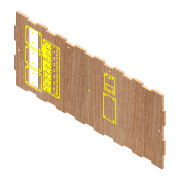
# Autodesk Inventor part: onderplaat elektrobix v2
Saved by Autodesk Inventor 2020.3 (Build 243373000, 373)
## iProperties
Created: 2020-11-25
Part Number: onderplaat elektrobix v2
Material: Wood (Birch)
Document SubType Name: Sheet Metal
Designer: Svend
Density: 0.55 g/cm^3
Sheet Metal Rule: Default_mm
Appearance: Birch - Natural Polished
Author: Svend
Autodesk Inventor part; units mm, degrees
(part 1 of 2)
ref_plane "YZ Plane" through (0, 0, 0) normal (1, 0, 0) x (0, 1, 0)
ref_plane "XZ Plane" through (0, 0, 0) normal (0, 1, 0) x (-1, 0, 0)
ref_plane "XY Plane" through (0, 0, 0) normal (0, 0, 1) x (1, 0, 0)
sketch "Sketch1" plane through (0, 0, 0) normal (0, 0, 1) x (1, 0, 0)
  line L0 (-235, 100) -> (235, 100)
  line L1 (235, 100) -> (235, -100)
  line L2 (235, -100) -> (-235, -100)
  line L3 (-235, -100) -> (-235, 100)
  line L4 (-235, 100) -> (235, -100) construction
  line L5 (235, 100) -> (-235, -100) construction
  line L6 (-15, 94) -> (15, 94)
  line L7 (15, 94) -> (15, 100)
  line L8 (15, 100) -> (-15, 100)
  line L9 (-15, 100) -> (-15, 94)
  line L10 (-15, 94) -> (15, 100) construction
  line L11 (15, 94) -> (-15, 100) construction
  line L12 (45, 94) -> (75, 94)
  line L13 (75, 94) -> (75, 100)
  line L14 (75, 100) -> (45, 100)
  line L15 (45, 100) -> (45, 94)
  line L16 (45, 94) -> (75, 100) construction
  line L17 (75, 94) -> (45, 100) construction
  line L18 (105, 94) -> (135, 94)
  line L19 (135, 94) -> (135, 100)
  line L20 (135, 100) -> (105, 100)
  line L21 (105, 100) -> (105, 94)
  line L22 (105, 94) -> (135, 100) construction
  line L23 (135, 94) -> (105, 100) construction
  line L24 (165, 94) -> (195, 94)
  line L25 (195, 94) -> (195, 100)
  line L26 (195, 100) -> (165, 100)
  line L27 (165, 100) -> (165, 94)
  line L28 (165, 94) -> (195, 100) construction
  line L29 (195, 94) -> (165, 100) construction
  line L30 (-75, 94) -> (-45, 94)
  line L31 (-45, 94) -> (-45, 100)
  line L32 (-45, 100) -> (-75, 100)
  line L33 (-75, 100) -> (-75, 94)
  line L34 (-75, 94) -> (-45, 100) construction
  line L35 (-45, 94) -> (-75, 100) construction
  line L36 (-15, 94) -> (15, 94)
  line L37 (15, 94) -> (15, 100)
  line L38 (15, 100) -> (-15, 100)
  line L39 (-15, 100) -> (-15, 94)
  line L40 (-15, 94) -> (15, 100) construction
  line L41 (15, 94) -> (-15, 100) construction
  line L42 (45, 94) -> (75, 94)
  line L43 (75, 94) -> (75, 100)
  line L44 (75, 100) -> (45, 100)
  line L45 (45, 100) -> (45, 94)
  line L46 (45, 94) -> (75, 100) construction
  line L47 (75, 94) -> (45, 100) construction
  line L48 (105, 94) -> (135, 94)
  line L49 (135, 94) -> (135, 100)
  line L50 (135, 100) -> (105, 100)
  line L51 (105, 100) -> (105, 94)
  line L52 (105, 94) -> (135, 100) construction
  line L53 (135, 94) -> (105, 100) construction
  line L54 (-135, 94) -> (-105, 94)
  line L55 (-105, 94) -> (-105, 100)
  line L56 (-105, 100) -> (-135, 100)
  line L57 (-135, 100) -> (-135, 94)
  line L58 (-135, 94) -> (-105, 100) construction
  line L59 (-105, 94) -> (-135, 100) construction
  line L60 (-75, 94) -> (-45, 94)
  line L61 (-45, 94) -> (-45, 100)
  line L62 (-45, 100) -> (-75, 100)
  line L63 (-75, 100) -> (-75, 94)
  line L64 (-75, 94) -> (-45, 100) construction
  line L65 (-45, 94) -> (-75, 100) construction
  line L66 (-15, 94) -> (15, 94)
  line L67 (15, 94) -> (15, 100)
  line L68 (15, 100) -> (-15, 100)
  line L69 (-15, 100) -> (-15, 94)
  line L70 (-15, 94) -> (15, 100) construction
  line L71 (15, 94) -> (-15, 100) construction
  line L72 (45, 94) -> (75, 94)
  line L73 (75, 94) -> (75, 100)
  line L74 (75, 100) -> (45, 100)
  line L75 (45, 100) -> (45, 94)
  line L76 (45, 94) -> (75, 100) construction
  line L77 (75, 94) -> (45, 100) construction
  line L78 (-195, 94) -> (-165, 94)
  line L79 (-165, 94) -> (-165, 100)
  line L80 (-165, 100) -> (-195, 100)
  line L81 (-195, 100) -> (-195, 94)
  line L82 (-195, 94) -> (-165, 100) construction
  line L83 (-165, 94) -> (-195, 100) construction
  line L84 (-135, 94) -> (-105, 94)
  line L85 (-105, 94) -> (-105, 100)
  line L86 (-105, 100) -> (-135, 100)
  line L87 (-135, 100) -> (-135, 94)
  line L88 (-135, 94) -> (-105, 100) construction
  line L89 (-105, 94) -> (-135, 100) construction
  line L90 (-75, 94) -> (-45, 94)
  line L91 (-45, 94) -> (-45, 100)
  line L92 (-45, 100) -> (-75, 100)
  line L93 (-75, 100) -> (-75, 94)
  line L94 (-75, 94) -> (-45, 100) construction
  line L95 (-45, 94) -> (-75, 100) construction
  line L96 (-15, 94) -> (15, 94)
  line L97 (15, 94) -> (15, 100)
  line L98 (15, 100) -> (-15, 100)
  line L99 (-15, 100) -> (-15, 94)
  line L100 (-15, 94) -> (15, 100) construction
  line L101 (15, 94) -> (-15, 100) construction
  line L102 (229, -20) -> (235, -20)
  line L103 (235, -20) -> (235, 20)
  line L104 (235, 20) -> (229, 20)
  line L105 (229, 20) -> (229, -20)
  line L106 (229, -20) -> (235, 20) construction
  line L107 (235, -20) -> (229, 20) construction
  line L108 (235, 100) -> (229, 100)
  line L109 (229, 100) -> (229, 60)
  line L110 (229, 60) -> (235, 60)
  line L111 (235, 60) -> (235, 100)
  line L112 (235, -100) -> (229, -100)
  line L113 (229, -100) -> (229, -60)
  line L114 (229, -60) -> (235, -60)
  line L115 (235, -60) -> (235, -100)
  line L116 (0, 100) -> (0, -100) construction
  line L117 (235, 0) -> (-235, 0) construction
  line L118 (-229, -20) -> (-235, -20)
  line L119 (-235, -20) -> (-235, 20)
  line L120 (-235, 20) -> (-229, 20)
  line L121 (-229, 20) -> (-229, -20)
  line L122 (-229, -20) -> (-235, 20) construction
  line L123 (-235, -20) -> (-229, 20) construction
  line L124 (-235, 100) -> (-229, 100)
  line L125 (-229, 100) -> (-229, 60)
  line L126 (-229, 60) -> (-235, 60)
  line L127 (-235, 60) -> (-235, 100)
  line L128 (-235, -100) -> (-229, -100)
  line L129 (-229, -100) -> (-229, -60)
  line L130 (-229, -60) -> (-235, -60)
  line L131 (-235, -60) -> (-235, -100)
  line L132 (-15, -94) -> (15, -94)
  line L133 (15, -94) -> (15, -100)
  line L134 (15, -100) -> (-15, -100)
  line L135 (-15, -100) -> (-15, -94)
  line L136 (-15, -94) -> (15, -100) construction
  line L137 (15, -94) -> (-15, -100) construction
  line L138 (45, -100) -> (45, -94)
  line L139 (45, -94) -> (75, -94)
  line L140 (75, -100) -> (45, -100)
  line L141 (45, -94) -> (75, -100) construction
  line L142 (75, -94) -> (45, -100) construction
  line L143 (75, -94) -> (75, -100)
  line L144 (105, -100) -> (105, -94)
  line L145 (105, -94) -> (135, -94)
  line L146 (135, -100) -> (105, -100)
  line L147 (105, -94) -> (135, -100) construction
  line L148 (135, -94) -> (105, -100) construction
  line L149 (135, -94) -> (135, -100)
  line L150 (165, -100) -> (165, -94)
  line L151 (165, -94) -> (195, -94)
  line L152 (195, -100) -> (165, -100)
  line L153 (165, -94) -> (195, -100) construction
  line L154 (195, -94) -> (165, -100) construction
  line L155 (195, -94) -> (195, -100)
  line L156 (-75, -100) -> (-75, -94)
  line L157 (-75, -94) -> (-45, -94)
  line L158 (-45, -100) -> (-75, -100)
  line L159 (-75, -94) -> (-45, -100) construction
  line L160 (-45, -94) -> (-75, -100) construction
  line L161 (-45, -94) -> (-45, -100)
  line L162 (-15, -100) -> (-15, -94)
  line L163 (-15, -94) -> (15, -94)
  line L164 (15, -100) -> (-15, -100)
  line L165 (-15, -94) -> (15, -100) construction
  line L166 (15, -94) -> (-15, -100) construction
  line L167 (15, -94) -> (15, -100)
  line L168 (45, -100) -> (45, -94)
  line L169 (45, -94) -> (75, -94)
  line L170 (75, -100) -> (45, -100)
  line L171 (45, -94) -> (75, -100) construction
  line L172 (75, -94) -> (45, -100) construction
  line L173 (75, -94) -> (75, -100)
  line L174 (105, -100) -> (105, -94)
  line L175 (105, -94) -> (135, -94)
  line L176 (135, -100) -> (105, -100)
  line L177 (105, -94) -> (135, -100) construction
  line L178 (135, -94) -> (105, -100) construction
  line L179 (135, -94) -> (135, -100)
  line L180 (-135, -100) -> (-135, -94)
  line L181 (-135, -94) -> (-105, -94)
  line L182 (-105, -100) -> (-135, -100)
  line L183 (-135, -94) -> (-105, -100) construction
  line L184 (-105, -94) -> (-135, -100) construction
  line L185 (-105, -94) -> (-105, -100)
  line L186 (-75, -100) -> (-75, -94)
  line L187 (-75, -94) -> (-45, -94)
  line L188 (-45, -100) -> (-75, -100)
  line L189 (-75, -94) -> (-45, -100) construction
  line L190 (-45, -94) -> (-75, -100) construction
  line L191 (-45, -94) -> (-45, -100)
  line L192 (-15, -100) -> (-15, -94)
  line L193 (-15, -94) -> (15, -94)
  line L194 (15, -100) -> (-15, -100)
  line L195 (-15, -94) -> (15, -100) construction
  line L196 (15, -94) -> (-15, -100) construction
  line L197 (15, -94) -> (15, -100)
  line L198 (45, -100) -> (45, -94)
  line L199 (45, -94) -> (75, -94)
  line L200 (75, -100) -> (45, -100)
  line L201 (45, -94) -> (75, -100) construction
  line L202 (75, -94) -> (45, -100) construction
  line L203 (75, -94) -> (75, -100)
  line L204 (-195, -100) -> (-195, -94)
  line L205 (-195, -94) -> (-165, -94)
  line L206 (-165, -100) -> (-195, -100)
  line L207 (-195, -94) -> (-165, -100) construction
  line L208 (-165, -94) -> (-195, -100) construction
  line L209 (-165, -94) -> (-165, -100)
  line L210 (-135, -100) -> (-135, -94)
  line L211 (-135, -94) -> (-105, -94)
  line L212 (-105, -100) -> (-135, -100)
  line L213 (-135, -94) -> (-105, -100) construction
  line L214 (-105, -94) -> (-135, -100) construction
  line L215 (-105, -94) -> (-105, -100)
  line L216 (-75, -100) -> (-75, -94)
  line L217 (-75, -94) -> (-45, -94)
  line L218 (-45, -100) -> (-75, -100)
  line L219 (-75, -94) -> (-45, -100) construction
  line L220 (-45, -94) -> (-75, -100) construction
  line L221 (-45, -94) -> (-45, -100)
  line L222 (-15, -100) -> (-15, -94)
  line L223 (-15, -94) -> (15, -94)
  line L224 (15, -100) -> (-15, -100)
  line L225 (-15, -94) -> (15, -100) construction
  line L226 (15, -94) -> (-15, -100) construction
  line L227 (15, -94) -> (15, -100)
  circle A0 centre (-65, 85) radius 3
  circle A1 centre (65, 85) radius 3
  line L228 (65, 85) -> (-65, 85) construction
  circle A2 centre (-220, 0) radius 3
  circle A3 centre (220, 0) radius 3
  point P0 (0, 0)
  point P1 (0, 97)
  point P2 (0, 97)
  point P3 (0, 0)
  point P4 (60, 97)
  point P5 (60, 97)
  point P6 (120, 97)
  point P7 (120, 97)
  point P8 (180, 97)
  point P9 (180, 97)
  point P10 (-60, 97)
  point P11 (-60, 97)
  point P12 (0, 97)
  point P13 (0, 97)
  point P14 (60, 97)
  point P15 (60, 97)
  point P16 (120, 97)
  point P17 (120, 97)
  point P18 (-120, 97)
  point P19 (-120, 97)
  point P20 (-60, 97)
  point P21 (-60, 97)
  point P22 (0, 97)
  point P23 (0, 97)
  point P24 (60, 97)
  point P25 (60, 97)
  point P26 (-180, 97)
  point P27 (-180, 97)
  point P28 (-120, 97)
  point P29 (-120, 97)
  point P30 (-60, 97)
  point P31 (-60, 97)
  point P32 (0, 97)
  point P33 (0, 97)
  point P34 (232, 0)
  point P35 (232, 0)
  point P36 (0, 0)
  point P37 (-232, 0)
  point P38 (-232, 0)
  point P39 (0, -97)
  point P40 (60, -100)
  point P41 (60, -97)
  point P42 (120, -100)
  point P43 (120, -97)
  point P44 (180, -100)
  point P45 (180, -97)
  point P46 (-60, -100)
  point P47 (-60, -97)
  point P48 (0, -97)
  point P49 (60, -100)
  point P50 (60, -97)
  point P51 (120, -100)
  point P52 (120, -97)
  point P53 (-120, -100)
  point P54 (-120, -97)
  point P55 (-60, -100)
  point P56 (-60, -97)
  point P57 (0, -97)
  point P58 (60, -100)
  point P59 (60, -97)
  point P60 (-180, -100)
  point P61 (-180, -97)
  point P62 (-120, -100)
  point P63 (-120, -97)
  point P64 (-60, -100)
  point P65 (-60, -97)
  point P66 (0, -97)
  point P67 (0, 85)
  point P68 (0, 100)
  dimension "d0" = 470
  dimension "d1" = 200
  dimension "d2" = 6
  dimension "d3" = 30
  dimension "d6" = 60
  dimension "d9" = 60
  dimension "d12" = 6
  dimension "d13" = 40
  dimension "d14" = 6
  dimension "d15" = 40
  dimension "d16" = 6
  dimension "d17" = 40
  dimension "d20" = 60
  dimension "d23" = 60
  dimension "d26" = 6
  dimension "d27" = 15
  dimension "d28" = 130
  dimension "d29" = 6
  dimension "d30" = 6
  dimension "d31" = 15
  dimension "d32" = 15
  measures "d0" distance of L1.end L2.end
  measures "d1" distance of L0.end L1.end
  measures "d2" distance of L6.end L7.end
  measures "d3" distance of L6.start L6.end
  measures "d6" distance of L6.start L12.start
  measures "d9" distance of L6.start L30.start
  measures "d12" distance of L103.end L104.end
  measures "d13" distance of L104.end L102.start
  measures "d14" distance of L110.end L109.end
  measures "d15" distance of L109.end L108.end
  measures "d16" distance of L113.end L114.end
  measures "d17" distance of L112.end L113.end
  measures "d20" distance of L116.end point (60, -100)
  measures "d23" distance of L116.end point (-60, -100)
  measures "d26" diameter of A1
  measures "d27" distance between parallel lines of L0 L228
  measures "d28" distance of L228.start L228.end
  measures "d29" diameter of A2
  measures "d30" diameter of A3
  measures "d31" distance from line of L3 A2.centre
  measures "d32" distance from line of L103 A3.centre
extrude "Plate1" add sketch "Sketch1" along normal blind 6 contours L0 L81 L78 L79 L57 L54 L55 L33 L30 L31 L9 L6 L7 L15 L12 L13 L21 L18 L19 L27 L24 L25 L109 L110 L1 L104 L105 L102 L114 L113 L2 L155 L151 L150 L149 L145 L144 L143 L139 L138 L133 L132 L135 L161 L157 L156 L185 L181 L180 L209 L205 L204 L129 L130 L3 L118 L121 L120 L126 L125
sketch "Sketch2" plane through (0, 0, 0) normal (0, 0, -1) x (-1, 0, 0)
  line L0 (160, -80) -> (193, -80)
  line L1 (193, -80) -> (193, 80)
  line L2 (193, 80) -> (160, 80)
  line L3 (160, 80) -> (160, -80)
  circle A0 centre (65, 85) radius 3 projected
  circle A1 centre (-65, 85) radius 3 projected
  circle A2 centre (220, 0) radius 3 projected
  circle A3 centre (-220, 0) radius 3 projected
  line L4 (235, -20) -> (229, -20) projected
  line L5 (229, -20) -> (229, 20) projected
  line L6 (229, 20) -> (235, 20) projected
  line L7 (235, 60) -> (235, 20) projected
  line L8 (235, 60) -> (229, 60) projected
  line L9 (229, 60) -> (229, 100) projected
  line L10 (195, 100) -> (229, 100) projected
  line L11 (195, 100) -> (195, 94) projected
  line L12 (195, 94) -> (165, 94) projected
  line L13 (165, 94) -> (165, 100) projected
  line L14 (135, 100) -> (165, 100) projected
  line L15 (135, 100) -> (135, 94) projected
  line L16 (135, 94) -> (105, 94) projected
  line L17 (105, 94) -> (105, 100) projected
  line L18 (75, 100) -> (105, 100) projected
  line L19 (75, 100) -> (75, 94) projected
  line L20 (75, 94) -> (45, 94) projected
  line L21 (45, 94) -> (45, 100) projected
  line L22 (15, 100) -> (45, 100) projected
  line L23 (15, 100) -> (15, 94) projected
  line L24 (15, 94) -> (-15, 94) projected
  line L25 (-15, 94) -> (-15, 100) projected
  line L26 (-45, 100) -> (-15, 100) projected
  line L27 (-45, 100) -> (-45, 94) projected
  line L28 (-45, 94) -> (-75, 94) projected
  line L29 (-75, 94) -> (-75, 100) projected
  line L30 (-105, 100) -> (-75, 100) projected
  line L31 (-105, 100) -> (-105, 94) projected
  line L32 (-105, 94) -> (-135, 94) projected
  line L33 (-135, 94) -> (-135, 100) projected
  line L34 (-165, 100) -> (-135, 100) projected
  line L35 (-165, 100) -> (-165, 94) projected
  line L36 (-165, 94) -> (-195, 94) projected
  line L37 (-195, 94) -> (-195, 100) projected
  line L38 (-229, 100) -> (-195, 100) projected
  line L39 (-229, 100) -> (-229, 60) projected
  line L40 (-229, 60) -> (-235, 60) projected
  line L41 (-235, 20) -> (-235, 60) projected
  line L42 (-235, 20) -> (-229, 20) projected
  line L43 (-229, 20) -> (-229, -20) projected
  line L44 (-229, -20) -> (-235, -20) projected
  line L45 (-235, -60) -> (-235, -20) projected
  line L46 (-235, -60) -> (-229, -60) projected
  line L47 (-229, -60) -> (-229, -100) projected
  line L48 (-195, -100) -> (-229, -100) projected
  line L49 (-195, -100) -> (-195, -94) projected
  line L50 (-195, -94) -> (-165, -94) projected
  line L51 (-165, -94) -> (-165, -100) projected
  line L52 (-135, -100) -> (-165, -100) projected
  line L53 (-135, -100) -> (-135, -94) projected
  line L54 (-135, -94) -> (-105, -94) projected
  line L55 (-105, -94) -> (-105, -100) projected
  line L56 (-75, -100) -> (-105, -100) projected
  line L57 (-75, -100) -> (-75, -94) projected
  line L58 (-75, -94) -> (-45, -94) projected
  line L59 (-45, -94) -> (-45, -100) projected
  line L60 (-15, -100) -> (-45, -100) projected
  line L61 (-15, -100) -> (-15, -94) projected
  line L62 (-15, -94) -> (15, -94) projected
  line L63 (15, -94) -> (15, -100) projected
  line L64 (45, -100) -> (15, -100) projected
  line L65 (45, -100) -> (45, -94) projected
  line L66 (45, -94) -> (75, -94) projected
  line L67 (75, -94) -> (75, -100) projected
  line L68 (105, -100) -> (75, -100) projected
  line L69 (105, -100) -> (105, -94) projected
  line L70 (105, -94) -> (135, -94) projected
  line L71 (135, -94) -> (135, -100) projected
  line L72 (165, -100) -> (135, -100) projected
  line L73 (165, -100) -> (165, -94) projected
  line L74 (165, -94) -> (195, -94) projected
  line L75 (195, -94) -> (195, -100) projected
  line L76 (229, -100) -> (195, -100) projected
  line L77 (229, -100) -> (229, -60) projected
  line L78 (229, -60) -> (235, -60) projected
  line L79 (235, -20) -> (235, -60) projected
  point P0 (0, 0)
  point P1 (193, 0)
  point P2 (229, 0)
  dimension "d34" = 33
  dimension "d35" = 160
  dimension "d36" = 36
  constraints: 8 end point, 2 midpoint, 2 parallel, 1 horizontal, 1 horizontal alignment, 1 perpendicular
  measures "d34" distance of L2.end L1.end
  measures "d35" distance of L1.end L0.end
  measures "d36" distance between parallel lines of L5 L1
extrude "Cut1" cut sketch "Sketch2" against normal blind 6 contours L3 L2 L1 L0
sketch "Sketch3" plane through (0, 0, 6) normal (0, 0, 1) x (1, 0, 0)
  line L0 (-153.2, -29.5) -> (-195, -29.5)
  line L1 (-195, -29.5) -> (-199, -33.5)
  line L2 (-199, -33.5) -> (-199, -75)
  line L3 (-199, -75) -> (-195, -79)
  line L4 (-195, -79) -> (-153.2, -79)
  line L5 (-153.2, -79) -> (-149.2, -75)
  line L6 (-149.2, -75) -> (-149.2, -33.5)
  line L7 (-149.2, -33.5) -> (-153.2, -29.5)
  circle A0 centre (-176.5, -40.75) radius 1.6
  circle A1 centre (-176.5, -67.75) radius 1.6
  circle A2 centre (-195.4, -34.25) radius 1.6
  circle A3 centre (-195.4, -74.25) radius 1.6
  circle A4 centre (-155.4, -74.25) radius 1.6
  circle A5 centre (-155.4, -34.25) radius 1.6
  line L8 (-153.2, 25) -> (-195, 25)
  line L9 (-195, 25) -> (-199, 21)
  line L10 (-199, 21) -> (-199, -20.5)
  line L11 (-199, -20.5) -> (-195, -24.5)
  line L12 (-195, -24.5) -> (-153.2, -24.5)
  line L13 (-153.2, -24.5) -> (-149.2, -20.5)
  line L14 (-149.2, -20.5) -> (-149.2, 21)
  line L15 (-149.2, 21) -> (-153.2, 25)
  circle A6 centre (-176.5, 13.75) radius 1.6
  circle A7 centre (-176.5, -13.25) radius 1.6
  circle A8 centre (-195.4, 20.25) radius 1.6
  circle A9 centre (-195.4, -19.75) radius 1.6
  circle A10 centre (-155.4, -19.75) radius 1.6
  circle A11 centre (-155.4, 20.25) radius 1.6
  line L16 (-153.2, 79.5) -> (-195, 79.5)
  line L17 (-195, 79.5) -> (-199, 75.5)
  line L18 (-199, 75.5) -> (-199, 34)
  line L19 (-199, 34) -> (-195, 30)
  line L20 (-195, 30) -> (-153.2, 30)
  line L21 (-153.2, 30) -> (-149.2, 34)
  line L22 (-149.2, 34) -> (-149.2, 75.5)
  line L23 (-149.2, 75.5) -> (-153.2, 79.5)
  circle A12 centre (-176.5, 68.25) radius 1.6
  circle A13 centre (-176.5, 41.25) radius 1.6
  circle A14 centre (-195.4, 74.75) radius 1.6
  circle A15 centre (-195.4, 34.75) radius 1.6
  circle A16 centre (-155.4, 34.75) radius 1.6
  circle A17 centre (-155.4, 74.75) radius 1.6
  arc A18 (-96.55, -69) -> (-94, -66.45) centre (-96.55, -66.45) ccw
  line L24 (-94, -66.45) -> (-94, 66.45)
  arc A19 (-94, 66.45) -> (-96.55, 69) centre (-96.55, 66.45) ccw
  line L25 (-96.55, 69) -> (-141.45, 69)
  arc A20 (-141.45, 69) -> (-144, 66.45) centre (-141.45, 66.45) ccw
  line L26 (-144, 66.45) -> (-144, -66.45)
  arc A21 (-144, -66.45) -> (-141.45, -69) centre (-141.45, -66.45) ccw
  line L27 (-141.45, -69) -> (-96.55, -69)
  line L28 (-137, -48.3571) -> (-137, -42.7571)
  line L29 (-137, -42.7571) -> (-131, -42.7571)
  line L30 (-131, -42.7571) -> (-131, -48.3571)
  line L31 (-131, -48.3571) -> (-137, -48.3571)
  line L32 (-129.5, -38.6571) -> (-129.5, -38.3571)
  line L33 (-129.5, -38.3571) -> (-127.6, -38.3571)
  line L34 (-127.6, -38.3571) -> (-127.6, -37.6571)
  line L35 (-127.6, -37.6571) -> (-127.3, -37.6571)
  line L36 (-127.3, -37.6571) -> (-127.3, -38.6571)
  line L37 (-127.3, -38.6571) -> (-129.5, -38.6571)
  line L38 (-138.3, 8.9714) -> (-138.3, 14.1714)
  line L39 (-138.3, 14.1714) -> (-135.7, 14.1714)
  line L40 (-135.7, 14.1714) -> (-135.7, 8.9714)
  line L41 (-135.7, 8.9714) -> (-138.3, 8.9714)
  line L42 (-128.7, 7.9714) -> (-126, 7.9714)
  line L43 (-126, 7.9714) -> (-126, 10.3714)
  line L44 (-126, 10.3714) -> (-124.2, 12.1714)
  line L45 (-124.2, 12.1714) -> (-119.5, 12.1714)
  line L46 (-119.5, 12.1714) -> (-119.5, 11.0714)
  line L47 (-119.5, 11.0714) -> (-123.8858, 11.0714)
  line L48 (-123.8858, 11.0714) -> (-124.9, 10.0572)
  line L49 (-124.9, 10.0572) -> (-124.9, 6.2856)
  line L50 (-124.9, 6.2856) -> (-123.8858, 5.2714)
  line L51 (-123.8858, 5.2714) -> (-119.5, 5.2714)
  line L52 (-119.5, 5.2714) -> (-119.5, 4.1714)
  line L53 (-119.5, 4.1714) -> (-124.2, 4.1714)
  line L54 (-124.2, 4.1714) -> (-126, 5.9714)
  line L55 (-126, 5.9714) -> (-126, 1.2714)
  line L56 (-126, 1.2714) -> (-128.7, 1.2714)
  line L57 (-128.7, 1.2714) -> (-128.7, 7.9714)
  line L58 (-138.3, 42.0571) -> (-138.3, 47.2571)
  line L59 (-138.3, 47.2571) -> (-135.7, 47.2571)
  line L60 (-135.7, 47.2571) -> (-135.7, 42.0571)
  line L61 (-135.7, 42.0571) -> (-138.3, 42.0571)
  line L62 (-135.5, 47.2571) -> (-133.2, 47.2571)
  line L63 (-133.2, 47.2571) -> (-133.2, 42.0571)
  line L64 (-133.2, 42.0571) -> (-135.5, 42.0571)
  line L65 (-135.5, 42.0571) -> (-135.5, 47.2571)
  line L66 (-128.7, 41.0571) -> (-126, 41.0571)
  line L67 (-126, 41.0571) -> (-126, 43.4571)
  line L68 (-126, 43.4571) -> (-124.2, 45.2571)
  line L69 (-124.2, 45.2571) -> (-119.5, 45.2571)
  line L70 (-119.5, 45.2571) -> (-119.5, 44.1571)
  line L71 (-119.5, 44.1571) -> (-123.8858, 44.1571)
  line L72 (-123.8858, 44.1571) -> (-124.9, 43.1429)
  line L73 (-124.9, 43.1429) -> (-124.9, 39.3714)
  line L74 (-124.9, 39.3714) -> (-123.8858, 38.3571)
  line L75 (-123.8858, 38.3571) -> (-119.5, 38.3571)
  line L76 (-119.5, 38.3571) -> (-119.5, 37.2571)
  line L77 (-119.5, 37.2571) -> (-124.2, 37.2571)
  line L78 (-124.2, 37.2571) -> (-126, 39.0571)
  line L79 (-126, 39.0571) -> (-126, 34.3571)
  line L80 (-126, 34.3571) -> (-128.7, 34.3571)
  line L81 (-128.7, 34.3571) -> (-128.7, 41.0571)
  line L82 (-128.7, 24.5143) -> (-126, 24.5143)
  line L83 (-126, 24.5143) -> (-126, 26.9143)
  line L84 (-126, 26.9143) -> (-124.2, 28.7143)
  line L85 (-124.2, 28.7143) -> (-119.5, 28.7143)
  line L86 (-119.5, 28.7143) -> (-119.5, 27.6143)
  line L87 (-119.5, 27.6143) -> (-123.8858, 27.6143)
  line L88 (-123.8858, 27.6143) -> (-124.9, 26.6001)
  line L89 (-124.9, 26.6001) -> (-124.9, 22.8285)
  line L90 (-124.9, 22.8285) -> (-123.8858, 21.8143)
  line L91 (-123.8858, 21.8143) -> (-119.5, 21.8143)
  line L92 (-119.5, 21.8143) -> (-119.5, 20.7143)
  line L93 (-119.5, 20.7143) -> (-124.2, 20.7143)
  line L94 (-124.2, 20.7143) -> (-126, 22.5143)
  line L95 (-126, 22.5143) -> (-126, 17.8143)
  line L96 (-126, 17.8143) -> (-128.7, 17.8143)
  line L97 (-128.7, 17.8143) -> (-128.7, 24.5143)
  line L98 (-133, 14.1714) -> (-130.7, 14.1714)
  line L99 (-130.7, 14.1714) -> (-130.7, 8.9714)
  line L100 (-130.7, 8.9714) -> (-133, 8.9714)
  line L101 (-133, 8.9714) -> (-133, 14.1714)
  line L102 (-135.5, -18.9143) -> (-133.2, -18.9143)
  line L103 (-133.2, -18.9143) -> (-133.2, -24.1143)
  line L104 (-133.2, -24.1143) -> (-135.5, -24.1143)
  line L105 (-135.5, -24.1143) -> (-135.5, -18.9143)
  line L106 (-133, -52) -> (-130.7, -52)
  line L107 (-130.7, -52) -> (-130.7, -57.2)
  line L108 (-130.7, -57.2) -> (-133, -57.2)
  line L109 (-133, -57.2) -> (-133, -52)
  line L110 (-138.3, -40.6571) -> (-138.3, -35.4571)
  line L111 (-138.3, -35.4571) -> (-135.7, -35.4571)
  line L112 (-135.7, -35.4571) -> (-135.7, -40.6571)
  line L113 (-135.7, -40.6571) -> (-138.3, -40.6571)
  line L114 (-127.3, -35.4571) -> (-127.3, -36.4571)
  line L115 (-127.3, -36.4571) -> (-127.6, -36.4571)
  line L116 (-127.6, -36.4571) -> (-127.6, -35.7571)
  line L117 (-127.6, -35.7571) -> (-129.5, -35.7571)
  line L118 (-129.5, -35.7571) -> (-129.5, -35.4571)
  line L119 (-129.5, -35.4571) -> (-127.3, -35.4571)
  line L120 (-137, -15.2714) -> (-137, -9.6714)
  line L121 (-137, -9.6714) -> (-131, -9.6714)
  line L122 (-131, -9.6714) -> (-131, -15.2714)
  line L123 (-131, -15.2714) -> (-137, -15.2714)
  line L124 (-135.5, 14.1714) -> (-133.2, 14.1714)
  line L125 (-133.2, 14.1714) -> (-133.2, 8.9714)
  line L126 (-133.2, 8.9714) -> (-135.5, 8.9714)
  line L127 (-135.5, 8.9714) -> (-135.5, 14.1714)
  line L128 (-129.5, 10.9714) -> (-129.5, 11.2714)
  line L129 (-129.5, 11.2714) -> (-127.6, 11.2714)
  line L130 (-127.6, 11.2714) -> (-127.6, 11.9714)
  line L131 (-127.6, 11.9714) -> (-127.3, 11.9714)
  line L132 (-127.3, 11.9714) -> (-127.3, 10.9714)
  line L133 (-127.3, 10.9714) -> (-129.5, 10.9714)
  line L134 (-138.3, 63.8) -> (-135.7, 63.8)
  line L135 (-135.7, 63.8) -> (-135.7, 58.6)
  line L136 (-135.7, 58.6) -> (-138.3, 58.6)
  line L137 (-138.3, 58.6) -> (-138.3, 63.8)
  line L138 (-137, 56.5) -> (-131, 56.5)
  line L139 (-131, 56.5) -> (-131, 50.9)
  line L140 (-131, 50.9) -> (-137, 50.9)
  line L141 (-137, 50.9) -> (-137, 56.5)
  line L142 (-127.3, 63.8) -> (-127.3, 62.8)
  line L143 (-127.3, 62.8) -> (-127.6, 62.8)
  line L144 (-127.6, 62.8) -> (-127.6, 63.5)
  line L145 (-127.6, 63.5) -> (-129.5, 63.5)
  line L146 (-129.5, 63.5) -> (-129.5, 63.8)
  line L147 (-129.5, 63.8) -> (-127.3, 63.8)
  line L148 (-137, 34.3571) -> (-137, 39.9571)
  line L149 (-137, 39.9571) -> (-131, 39.9571)
  line L150 (-131, 39.9571) -> (-131, 34.3571)
  line L151 (-131, 34.3571) -> (-137, 34.3571)
  line L152 (-137, 1.2714) -> (-137, 6.8714)
  line L153 (-137, 6.8714) -> (-131, 6.8714)
  line L154 (-131, 6.8714) -> (-131, 1.2714)
  line L155 (-131, 1.2714) -> (-137, 1.2714)
  line L156 (-138.3, -24.1143) -> (-138.3, -18.9143)
  line L157 (-138.3, -18.9143) -> (-135.7, -18.9143)
  line L158 (-135.7, -18.9143) -> (-135.7, -24.1143)
  line L159 (-135.7, -24.1143) -> (-138.3, -24.1143)
  line L160 (-135.5, -52) -> (-133.2, -52)
  line L161 (-133.2, -52) -> (-133.2, -57.2)
  line L162 (-133.2, -57.2) -> (-135.5, -57.2)
  line L163 (-135.5, -57.2) -> (-135.5, -52)
  circle A22 centre (-137.8, -63.36) radius 0.6
  line L164 (-130.3, -53.4) -> (-130.3, -52.5)
  line L165 (-130.3, -52.5) -> (-129.7, -52.5)
  line L166 (-129.7, -52.5) -> (-129.7, -53.4)
  line L167 (-129.7, -53.4) -> (-130.3, -53.4)
  circle A23 centre (-137.8, -44.2771) radius 0.6
  circle A24 centre (-130.18, -30.2743) radius 0.6
  line L168 (-127.9, -20.9643) -> (-127.9, -20.0643)
  line L169 (-127.9, -20.0643) -> (-127.3, -20.0643)
  line L170 (-127.3, -20.0643) -> (-127.3, -20.9643)
  line L171 (-127.3, -20.9643) -> (-127.9, -20.9643)
  circle A25 centre (-130.18, -11.1914) radius 0.6
  line L172 (-130.3, -5.0714) -> (-130.3, -4.1714)
  line L173 (-130.3, -4.1714) -> (-129.7, -4.1714)
  line L174 (-129.7, -4.1714) -> (-129.7, -5.0714)
  line L175 (-129.7, -5.0714) -> (-130.3, -5.0714)
  circle A26 centre (-137.8, 2.8114) radius 0.6
  line L176 (-130.3, 12.7714) -> (-130.3, 13.6714)
  line L177 (-130.3, 13.6714) -> (-129.7, 13.6714)
  line L178 (-129.7, 13.6714) -> (-129.7, 12.7714)
  line L179 (-129.7, 12.7714) -> (-130.3, 12.7714)
  circle A27 centre (-137.8, 21.8943) radius 0.6
  circle A28 centre (-130.18, 35.8971) radius 0.6
  line L180 (-127.9, 45.2071) -> (-127.9, 46.1071)
  line L181 (-127.9, 46.1071) -> (-127.3, 46.1071)
  line L182 (-127.3, 46.1071) -> (-127.3, 45.2071)
  line L183 (-127.3, 45.2071) -> (-127.9, 45.2071)
  circle A29 centre (-137.8, 52.44) radius 0.6
  circle A30 centre (-130.18, 52.44) radius 0.6
  line L184 (-127.3, 61.75) -> (-127.9, 61.75)
  line L185 (-127.9, 61.75) -> (-127.9, 62.65)
  line L186 (-127.9, 62.65) -> (-127.3, 62.65)
  line L187 (-127.3, 62.65) -> (-127.3, 61.75)
  circle A31 centre (-137.8, 38.4371) radius 0.6
  line L188 (-130.3, 29.3143) -> (-130.3, 30.2143)
  line L189 (-130.3, 30.2143) -> (-129.7, 30.2143)
  line L190 (-129.7, 30.2143) -> (-129.7, 29.3143)
  line L191 (-129.7, 29.3143) -> (-130.3, 29.3143)
  circle A32 centre (-137.8, 19.3543) radius 0.6
  line L192 (-130.3, 11.4714) -> (-130.3, 12.3714)
  line L193 (-130.3, 12.3714) -> (-129.7, 12.3714)
  line L194 (-129.7, 12.3714) -> (-129.7, 11.4714)
  line L195 (-129.7, 11.4714) -> (-130.3, 11.4714)
  circle A33 centre (-130.18, 5.3514) radius 0.6
  line L196 (-127.9, -4.4214) -> (-127.9, -3.5214)
  line L197 (-127.9, -3.5214) -> (-127.3, -3.5214)
  line L198 (-127.3, -3.5214) -> (-127.3, -4.4214)
  line L199 (-127.3, -4.4214) -> (-127.9, -4.4214)
  circle A34 centre (-130.18, -13.7314) radius 0.6
  circle A35 centre (-137.8, -27.7343) radius 0.6
  line L200 (-127.9, -37.5071) -> (-127.9, -36.6071)
  line L201 (-127.9, -36.6071) -> (-127.3, -36.6071)
  line L202 (-127.3, -36.6071) -> (-127.3, -37.5071)
  line L203 (-127.3, -37.5071) -> (-127.9, -37.5071)
  circle A36 centre (-137.8, -46.8171) radius 0.6
  line L204 (-130.3, -54.7) -> (-130.3, -53.8)
  line L205 (-130.3, -53.8) -> (-129.7, -53.8)
  line L206 (-129.7, -53.8) -> (-129.7, -54.7)
  line L207 (-129.7, -54.7) -> (-130.3, -54.7)
  circle A37 centre (-130.18, -60.82) radius 0.6
  circle A38 centre (-137.8, -60.82) radius 0.6
  circle A39 centre (-130.18, -46.8171) radius 0.6
  line L208 (-130.3, -38.1571) -> (-130.3, -37.2571)
  line L209 (-130.3, -37.2571) -> (-129.7, -37.2571)
  line L210 (-129.7, -37.2571) -> (-129.7, -38.1571)
  line L211 (-129.7, -38.1571) -> (-130.3, -38.1571)
  circle A40 centre (-130.18, -27.7343) radius 0.6
  line L212 (-130.3, -21.6143) -> (-130.3, -20.7143)
  line L213 (-130.3, -20.7143) -> (-129.7, -20.7143)
  line L214 (-129.7, -20.7143) -> (-129.7, -21.6143)
  line L215 (-129.7, -21.6143) -> (-130.3, -21.6143)
  circle A41 centre (-137.8, -13.7314) radius 0.6
  line L216 (-130.3, -3.7714) -> (-130.3, -2.8714)
  line L217 (-130.3, -2.8714) -> (-129.7, -2.8714)
  line L218 (-129.7, -2.8714) -> (-129.7, -3.7714)
  line L219 (-129.7, -3.7714) -> (-130.3, -3.7714)
  circle A42 centre (-137.8, 5.3514) radius 0.6
  circle A43 centre (-130.18, 19.3543) radius 0.6
  line L220 (-127.9, 28.6643) -> (-127.9, 29.5643)
  line L221 (-127.9, 29.5643) -> (-127.3, 29.5643)
  line L222 (-127.3, 29.5643) -> (-127.3, 28.6643)
  line L223 (-127.3, 28.6643) -> (-127.9, 28.6643)
  circle A44 centre (-130.18, 38.4371) radius 0.6
  line L224 (-130.3, 44.5571) -> (-130.3, 45.4571)
  line L225 (-130.3, 45.4571) -> (-129.7, 45.4571)
  line L226 (-129.7, 45.4571) -> (-129.7, 44.5571)
  line L227 (-129.7, 44.5571) -> (-130.3, 44.5571)
  line L228 (-130.3, 62) -> (-129.7, 62)
  line L229 (-129.7, 62) -> (-129.7, 61.1)
  line L230 (-129.7, 61.1) -> (-130.3, 61.1)
  line L231 (-130.3, 61.1) -> (-130.3, 62)
  circle A45 centre (-137.8, 54.98) radius 0.6
  circle A46 centre (-130.18, 54.98) radius 0.6
  line L232 (-130.3, 63.3) -> (-129.7, 63.3)
  line L233 (-129.7, 63.3) -> (-129.7, 62.4)
  line L234 (-129.7, 62.4) -> (-130.3, 62.4)
  line L235 (-130.3, 62.4) -> (-130.3, 63.3)
  line L236 (-130.3, 45.8571) -> (-130.3, 46.7571)
  line L237 (-130.3, 46.7571) -> (-129.7, 46.7571)
  line L238 (-129.7, 46.7571) -> (-129.7, 45.8571)
  line L239 (-129.7, 45.8571) -> (-130.3, 45.8571)
  circle A47 centre (-137.8, 35.8971) radius 0.6
  line L240 (-130.3, 28.0143) -> (-130.3, 28.9143)
  line L241 (-130.3, 28.9143) -> (-129.7, 28.9143)
  line L242 (-129.7, 28.9143) -> (-129.7, 28.0143)
  line L243 (-129.7, 28.0143) -> (-130.3, 28.0143)
  circle A48 centre (-130.18, 21.8943) radius 0.6
  line L244 (-127.9, 12.1214) -> (-127.9, 13.0214)
  line L245 (-127.9, 13.0214) -> (-127.3, 13.0214)
  line L246 (-127.3, 13.0214) -> (-127.3, 12.1214)
  line L247 (-127.3, 12.1214) -> (-127.9, 12.1214)
  circle A49 centre (-130.18, 2.8114) radius 0.6
  circle A50 centre (-137.8, -11.1914) radius 0.6
  line L248 (-130.3, -20.3143) -> (-130.3, -19.4143)
  line L249 (-130.3, -19.4143) -> (-129.7, -19.4143)
  line L250 (-129.7, -19.4143) -> (-129.7, -20.3143)
  line L251 (-129.7, -20.3143) -> (-130.3, -20.3143)
  circle A51 centre (-137.8, -30.2743) radius 0.6
  line L252 (-130.3, -36.8571) -> (-130.3, -35.9571)
  line L253 (-130.3, -35.9571) -> (-129.7, -35.9571)
  line L254 (-129.7, -35.9571) -> (-129.7, -36.8571)
  line L255 (-129.7, -36.8571) -> (-130.3, -36.8571)
  circle A52 centre (-130.18, -44.2771) radius 0.6
  line L256 (-127.9, -54.05) -> (-127.9, -53.15)
  line L257 (-127.9, -53.15) -> (-127.3, -53.15)
  line L258 (-127.3, -53.15) -> (-127.3, -54.05)
  line L259 (-127.3, -54.05) -> (-127.9, -54.05)
  circle A53 centre (-130.18, -63.36) radius 0.6
  spline S0 degree 3 poles (-140.7827, 50.4646) (-140.7091, 50.5548) (-140.5859, 50.7055) (-140.4309, 50.8228) (-140.3687, 50.8699) knots 0 0 0 0 0.598214 1 1 1 1
  spline S1 degree 3 poles (-140.3687, 50.8699) (-140.3167, 50.8964) (-140.2146, 50.9483) (-140.1004, 50.9566) (-140.0445, 50.9607) knots 0 0 0 0 0.509636 1 1 1 1
  spline S2 degree 3 poles (-140.0445, 50.9607) (-139.961, 50.9519) (-139.7914, 50.9339) (-139.6645, 50.8196) (-139.6001, 50.7615) knots 0 0 0 0 0.491932 1 1 1 1
  spline S3 degree 3 poles (-139.6001, 50.7615) (-139.5458, 50.687) (-139.431, 50.5297) (-139.4196, 50.3348) (-139.4136, 50.2322) knots 0 0 0 0 0.473646 1 1 1 1
  spline S4 degree 3 poles (-139.4136, 50.2322) (-139.4191, 50.1327) (-139.4295, 49.9442) (-139.5368, 49.7896) (-139.5874, 49.7166) knots 0 0 0 0 0.527918 1 1 1 1
  spline S5 degree 3 poles (-139.5874, 49.7166) (-139.6455, 49.6596) (-139.7567, 49.5508) (-139.9105, 49.5308) (-139.9839, 49.5212) knots 0 0 0 0 0.522906 1 1 1 1
  spline S6 degree 3 poles (-139.9839, 49.5212) (-140.035, 49.5266) (-140.1439, 49.5381) (-140.2372, 49.596) (-140.2866, 49.6267) knots 0 0 0 0 0.46934 1 1 1 1
  spline S7 degree 3 poles (-140.2866, 49.6267) (-140.3449, 49.679) (-140.4876, 49.807) (-140.5896, 49.9698) (-140.6499, 50.0662) knots 0 0 0 0 0.408278 1 1 1 1
  spline S8 degree 3 poles (-140.6499, 50.0662) (-140.7257, 49.9678) (-140.8519, 49.8038) (-141.0062, 49.6662) (-141.0679, 49.6111) knots 0 0 0 0 0.599891 1 1 1 1
  spline S9 degree 3 poles (-141.0679, 49.6111) (-141.1339, 49.5678) (-141.262, 49.4839) (-141.4141, 49.4696) (-141.4878, 49.4627) knots 0 0 0 0 0.515962 1 1 1 1
  spline S10 degree 3 poles (-141.4878, 49.4627) (-141.5779, 49.4719) (-141.7602, 49.4907) (-141.8964, 49.6135) (-141.9654, 49.6755) knots 0 0 0 0 0.494223 1 1 1 1
  spline S11 degree 3 poles (-141.9654, 49.6755) (-142.0231, 49.7546) (-142.1445, 49.9206) (-142.157, 50.1263) (-142.1636, 50.2341) knots 0 0 0 0 0.476086 1 1 1 1
  spline S12 degree 3 poles (-142.1636, 50.2341) (-142.1559, 50.3509) (-142.1411, 50.5734) (-141.9961, 50.742) (-141.9273, 50.822) knots 0 0 0 0 0.524774 1 1 1 1
  spline S13 degree 3 poles (-141.9273, 50.822) (-141.864, 50.871) (-141.7414, 50.9658) (-141.5876, 50.9821) (-141.5132, 50.99) knots 0 0 0 0 0.51651 1 1 1 1
  spline S14 degree 3 poles (-141.5132, 50.99) (-141.4535, 50.9842) (-141.3283, 50.9721) (-141.2208, 50.9063) (-141.1646, 50.8718) knots 0 0 0 0 0.476673 1 1 1 1
  spline S15 degree 3 poles (-141.1646, 50.8718) (-141.1019, 50.8202) (-140.9572, 50.7011) (-140.8458, 50.5501) (-140.7827, 50.4646) knots 0 0 0 0 0.433546 1 1 1 1
  spline S16 degree 3 poles (-141.8589, 41.5388) (-141.9167, 41.6123) (-142.0044, 41.7236) (-142.0794, 41.8437) (-142.105, 41.8845) knots 0 0 0 0 0.659633 1 1 1 1
  spline S17 degree 3 poles (-142.105, 41.8845) (-142.1192, 41.9204) (-142.1479, 41.9926) (-142.1518, 42.0701) (-142.1538, 42.1091) knots 0 0 0 0 0.496788 1 1 1 1
  spline S18 degree 3 poles (-142.1538, 42.1091) (-142.1489, 42.1679) (-142.1392, 42.2835) (-142.0639, 42.3715) (-142.0269, 42.4148) knots 0 0 0 0 0.508469 1 1 1 1
  spline S19 degree 3 poles (-142.0269, 42.4148) (-141.9797, 42.4498) (-141.8808, 42.5233) (-141.7575, 42.5309) (-141.6929, 42.5349) knots 0 0 0 0 0.476477 1 1 1 1
  spline S20 degree 3 poles (-141.6929, 42.5349) (-141.6514, 42.5329) (-141.5718, 42.529) (-141.5005, 42.4934) (-141.4663, 42.4763) knots 0 0 0 0 0.52029 1 1 1 1
  spline S21 degree 3 poles (-141.4663, 42.4763) (-141.4211, 42.4419) (-141.3204, 42.3651) (-141.2533, 42.2574) (-141.2163, 42.198) knots 0 0 0 0 0.448989 1 1 1 1
  spline S22 degree 3 poles (-141.2163, 42.198) (-141.1715, 42.1107) (-141.062, 41.8974) (-140.9798, 41.672) (-140.9312, 41.5388) knots 0 0 0 0 0.409209 1 1 1 1
  line L260 (-140.9312, 41.5388) -> (-140.8609, 41.5388)
  spline S23 degree 3 poles (-140.8609, 41.5388) (-140.7838, 41.5388) (-140.6539, 41.5388) (-140.54, 41.5992) (-140.4937, 41.6238) knots 0 0 0 0 0.593366 1 1 1 1
  spline S24 degree 3 poles (-140.4937, 41.6238) (-140.4646, 41.6568) (-140.4028, 41.7272) (-140.3971, 41.821) (-140.3941, 41.8709) knots 0 0 0 0 0.469395 1 1 1 1
  spline S25 degree 3 poles (-140.3941, 41.8709) (-140.3961, 41.9089) (-140.3998, 41.9805) (-140.4411, 42.0388) (-140.4605, 42.0662) knots 0 0 0 0 0.531201 1 1 1 1
  spline S26 degree 3 poles (-140.4605, 42.0662) (-140.4828, 42.0878) (-140.5256, 42.1293) (-140.5846, 42.1368) (-140.6128, 42.1404) knots 0 0 0 0 0.521012 1 1 1 1
  line L261 (-140.6128, 42.1404) -> (-140.7261, 42.1365)
  spline S27 degree 3 poles (-140.7261, 42.1365) (-140.7535, 42.1377) (-140.8043, 42.1399) (-140.8457, 42.169) (-140.8648, 42.1824) knots 0 0 0 0 0.540437 1 1 1 1
  spline S28 degree 3 poles (-140.8648, 42.1824) (-140.879, 42.1992) (-140.9083, 42.2338) (-140.9118, 42.2792) (-140.9136, 42.3025) knots 0 0 0 0 0.485541 1 1 1 1
  spline S29 degree 3 poles (-140.9136, 42.3025) (-140.9116, 42.3254) (-140.9077, 42.3704) (-140.8776, 42.4041) (-140.8628, 42.4207) knots 0 0 0 0 0.507733 1 1 1 1
  spline S30 degree 3 poles (-140.8628, 42.4207) (-140.8434, 42.434) (-140.8019, 42.4627) (-140.7512, 42.4652) (-140.7241, 42.4666) knots 0 0 0 0 0.465621 1 1 1 1
  spline S31 degree 3 poles (-140.7241, 42.4666) (-140.6677, 42.4574) (-140.545, 42.4373) (-140.4609, 42.3447) (-140.4155, 42.2947) knots 0 0 0 0 0.459879 1 1 1 1
  spline S32 degree 3 poles (-140.4155, 42.2947) (-140.3746, 42.2276) (-140.2846, 42.0801) (-140.2783, 41.9068) (-140.2749, 41.8123) knots 0 0 0 0 0.454711 1 1 1 1
  spline S33 degree 3 poles (-140.2749, 41.8123) (-140.277, 41.739) (-140.2808, 41.6039) (-140.3317, 41.4789) (-140.355, 41.4216) knots 0 0 0 0 0.54209 1 1 1 1
  spline S34 degree 3 poles (-140.355, 41.4216) (-140.3784, 41.3856) (-140.4263, 41.312) (-140.5045, 41.2721) (-140.5445, 41.2517) knots 0 0 0 0 0.490038 1 1 1 1
  spline S35 degree 3 poles (-140.5445, 41.2517) (-140.5869, 41.2416) (-140.6997, 41.2148) (-140.8158, 41.2159) (-140.8882, 41.2166) knots 0 0 0 0 0.376838 1 1 1 1
  line L262 (-140.8882, 41.2166) -> (-141.4956, 41.2166)
  spline S36 degree 3 poles (-141.4956, 41.2166) (-141.5644, 41.217) (-141.6691, 41.2177) (-141.7734, 41.2096) (-141.8091, 41.2068) knots 0 0 0 0 0.657591 1 1 1 1
  spline S37 degree 3 poles (-141.8091, 41.2068) (-141.8258, 41.2039) (-141.8541, 41.199) (-141.8769, 41.1817) (-141.8863, 41.1746) knots 0 0 0 0 0.588176 1 1 1 1
  spline S38 degree 3 poles (-141.8863, 41.1746) (-141.8919, 41.1668) (-141.9033, 41.1514) (-141.905, 41.1323) (-141.9058, 41.1228) knots 0 0 0 0 0.502185 1 1 1 1
  spline S39 degree 3 poles (-141.9058, 41.1228) (-141.9053, 41.1129) (-141.9044, 41.0937) (-141.8961, 41.0764) (-141.8921, 41.0681) knots 0 0 0 0 0.518564 1 1 1 1
  spline S40 degree 3 poles (-141.8921, 41.0681) (-141.8763, 41.0478) (-141.8326, 40.9917) (-141.7819, 40.9418) (-141.7495, 40.9099) knots 0 0 0 0 0.36168 1 1 1 1
  line L263 (-141.7495, 40.9099) -> (-141.8589, 40.9099)
  spline S41 degree 3 poles (-141.8589, 40.9099) (-141.9435, 40.9739) (-142.0879, 41.0832) (-142.1331, 41.2562) (-142.1519, 41.3279) knots 0 0 0 0 0.585755 1 1 1 1
  spline S42 degree 3 poles (-142.1519, 41.3279) (-142.1494, 41.3579) (-142.1446, 41.4164) (-142.1048, 41.4593) (-142.0855, 41.4802) knots 0 0 0 0 0.513246 1 1 1 1
  spline S43 degree 3 poles (-142.0855, 41.4802) (-142.0562, 41.4968) (-141.9863, 41.5362) (-141.9057, 41.5379) (-141.8589, 41.5388) knots 0 0 0 0 0.419859 1 1 1 1
  spline S44 degree 3 poles (-140.2749, 33.3455) (-140.2873, 33.2171) (-140.312, 32.9624) (-140.4935, 32.7824) (-140.5835, 32.6931) knots 0 0 0 0 0.504196 1 1 1 1
  spline S45 degree 3 poles (-140.5835, 32.6931) (-140.6749, 32.6322) (-140.8585, 32.5097) (-141.0785, 32.4927) (-141.189, 32.4841) knots 0 0 0 0 0.497855 1 1 1 1
  spline S46 degree 3 poles (-141.189, 32.4841) (-141.2705, 32.4895) (-141.439, 32.5007) (-141.5949, 32.5658) (-141.6753, 32.5994) knots 0 0 0 0 0.484054 1 1 1 1
  spline S47 degree 3 poles (-141.6753, 32.5994) (-141.7515, 32.6401) (-141.8986, 32.7188) (-141.9983, 32.8524) (-142.0464, 32.9168) knots 0 0 0 0 0.517802 1 1 1 1
  spline S48 degree 3 poles (-142.0464, 32.9168) (-142.0829, 32.9865) (-142.1566, 33.1276) (-142.1664, 33.2866) (-142.1714, 33.367) knots 0 0 0 0 0.494342 1 1 1 1
  spline S49 degree 3 poles (-142.1714, 33.367) (-142.1581, 33.4947) (-142.1316, 33.7495) (-141.9431, 33.923) (-141.8491, 34.0095) knots 0 0 0 0 0.501284 1 1 1 1
  spline S50 degree 3 poles (-141.8491, 34.0095) (-141.7559, 34.0682) (-141.5694, 34.1856) (-141.3496, 34.2023) (-141.2398, 34.2107) knots 0 0 0 0 0.500003 1 1 1 1
  spline S51 degree 3 poles (-141.2398, 34.2107) (-141.1569, 34.2051) (-140.9866, 34.1936) (-140.8306, 34.1242) (-140.7505, 34.0886) knots 0 0 0 0 0.486941 1 1 1 1
  spline S52 degree 3 poles (-140.7505, 34.0886) (-140.6757, 34.0463) (-140.5323, 33.9652) (-140.4368, 33.8313) (-140.3911, 33.7673) knots 0 0 0 0 0.521939 1 1 1 1
  spline S53 degree 3 poles (-140.3911, 33.7673) (-140.3572, 33.7003) (-140.2901, 33.5675) (-140.2799, 33.419) (-140.2749, 33.3455) knots 0 0 0 0 0.504638 1 1 1 1
  line L264 (-140.3277, 28.6521) -> (-141.4116, 28.6521)
  spline S54 degree 3 poles (-141.4116, 28.6521) (-141.4952, 28.6528) (-141.6221, 28.6539) (-141.7483, 28.6416) (-141.7915, 28.6375) knots 0 0 0 0 0.657959 1 1 1 1
  spline S55 degree 3 poles (-141.7915, 28.6375) (-141.812, 28.6328) (-141.848, 28.6245) (-141.8761, 28.6008) (-141.8882, 28.5906) knots 0 0 0 0 0.568313 1 1 1 1
  spline S56 degree 3 poles (-141.8882, 28.5906) (-141.8962, 28.5794) (-141.9122, 28.5568) (-141.9144, 28.5292) (-141.9155, 28.5154) knots 0 0 0 0 0.497728 1 1 1 1
  spline S57 degree 3 poles (-141.9155, 28.5154) (-141.9138, 28.4937) (-141.9099, 28.4464) (-141.892, 28.4024) (-141.8823, 28.3787) knots 0 0 0 0 0.459523 1 1 1 1
  line L265 (-141.8823, 28.3787) -> (-141.9507, 28.3513)
  line L266 (-141.9507, 28.3513) -> (-142.1714, 28.8865)
  line L267 (-142.1714, 28.8865) -> (-142.1714, 28.9744)
  line L268 (-142.1714, 28.9744) -> (-141.7925, 28.9744)
  spline S58 degree 3 poles (-141.7925, 28.9744) (-141.8636, 29.0393) (-141.9804, 29.1461) (-142.0713, 29.2753) (-142.107, 29.3259) knots 0 0 0 0 0.608228 1 1 1 1
  spline S59 degree 3 poles (-142.107, 29.3259) (-142.1258, 29.3668) (-142.1632, 29.448) (-142.1687, 29.5374) (-142.1714, 29.5818) knots 0 0 0 0 0.502321 1 1 1 1
  spline S60 degree 3 poles (-142.1714, 29.5818) (-142.1681, 29.6299) (-142.1615, 29.7244) (-142.1098, 29.8036) (-142.0845, 29.8425) knots 0 0 0 0 0.509274 1 1 1 1
  spline S61 degree 3 poles (-142.0845, 29.8425) (-142.0533, 29.8766) (-141.9907, 29.9449) (-141.9043, 29.9788) (-141.8609, 29.9959) knots 0 0 0 0 0.497322 1 1 1 1
  spline S62 degree 3 poles (-141.8609, 29.9959) (-141.8061, 30.0083) (-141.6789, 30.0373) (-141.5484, 30.0383) (-141.4741, 30.0388) knots 0 0 0 0 0.431063 1 1 1 1
  line L269 (-141.4741, 30.0388) -> (-140.6753, 30.0388)
  spline S63 degree 3 poles (-140.6753, 30.0388) (-140.6391, 30.0387) (-140.5788, 30.0385) (-140.5221, 30.0583) (-140.4995, 30.0662) knots 0 0 0 0 0.601307 1 1 1 1
  spline S64 degree 3 poles (-140.4995, 30.0662) (-140.4841, 30.0765) (-140.4527, 30.0977) (-140.4339, 30.1305) (-140.4243, 30.1472) knots 0 0 0 0 0.491054 1 1 1 1
  spline S65 degree 3 poles (-140.4243, 30.1472) (-140.4169, 30.1722) (-140.3979, 30.2354) (-140.3992, 30.3016) (-140.3999, 30.3416) knots 0 0 0 0 0.395508 1 1 1 1
  line L270 (-140.3999, 30.3416) -> (-140.3277, 30.3416)
  line L271 (-140.3277, 30.3416) -> (-140.3277, 29.7146)
  line L272 (-140.3277, 29.7146) -> (-141.5249, 29.7146)
  spline S66 degree 3 poles (-141.5249, 29.7146) (-141.5963, 29.7151) (-141.7149, 29.7159) (-141.8137, 29.6528) (-141.853, 29.6277) knots 0 0 0 0 0.602178 1 1 1 1
  spline S67 degree 3 poles (-141.853, 29.6277) (-141.8758, 29.5969) (-141.9221, 29.5345) (-141.9281, 29.457) (-141.9312, 29.4177) knots 0 0 0 0 0.492872 1 1 1 1
  spline S68 degree 3 poles (-141.9312, 29.4177) (-141.9283, 29.3875) (-141.922, 29.321) (-141.8938, 29.2603) (-141.8784, 29.2273) knots 0 0 0 0 0.455377 1 1 1 1
  spline S69 degree 3 poles (-141.8784, 29.2273) (-141.8541, 29.1875) (-141.7976, 29.095) (-141.7209, 29.0182) (-141.6773, 28.9744) knots 0 0 0 0 0.430104 1 1 1 1
  line L273 (-141.6773, 28.9744) -> (-140.6636, 28.9744)
  spline S70 degree 3 poles (-140.6636, 28.9744) (-140.6196, 28.9744) (-140.5452, 28.9745) (-140.483, 29.0139) (-140.4575, 29.03) knots 0 0 0 0 0.591253 1 1 1 1
  spline S71 degree 3 poles (-140.4575, 29.03) (-140.4418, 29.058) (-140.4017, 29.1292) (-140.4006, 29.2115) (-140.3999, 29.2615) knots 0 0 0 0 0.393373 1 1 1 1
  line L274 (-140.3999, 29.2615) -> (-140.3277, 29.2615)
  line L275 (-140.3277, 29.2615) -> (-140.3277, 28.6521)
  line L276 (-139.3394, 27.6052) -> (-141.7124, 27.6052)
  spline S72 degree 3 poles (-141.7124, 27.6052) (-141.7593, 27.6057) (-141.8347, 27.6064) (-141.9075, 27.5878) (-141.9351, 27.5808) knots 0 0 0 0 0.621846 1 1 1 1
  spline S73 degree 3 poles (-141.9351, 27.5808) (-141.9522, 27.5717) (-141.9861, 27.5535) (-142.0075, 27.5215) (-142.0181, 27.5056) knots 0 0 0 0 0.504 1 1 1 1
  spline S74 degree 3 poles (-142.0181, 27.5056) (-142.0263, 27.4816) (-142.047, 27.4204) (-142.0466, 27.3555) (-142.0464, 27.3162) knots 0 0 0 0 0.393301 1 1 1 1
  line L277 (-142.0464, 27.3162) -> (-142.1167, 27.3162)
  line L278 (-142.1167, 27.3162) -> (-142.1167, 28.1931)
  line L279 (-142.1167, 28.1931) -> (-142.0464, 28.1931)
  spline S75 degree 3 poles (-142.0464, 28.1931) (-142.0466, 28.1582) (-142.047, 28.1007) (-142.0283, 28.0465) (-142.021, 28.0252) knots 0 0 0 0 0.606784 1 1 1 1
  spline S76 degree 3 poles (-142.021, 28.0252) (-142.0107, 28.0108) (-141.9887, 27.9803) (-141.9549, 27.9636) (-141.937, 27.9548) knots 0 0 0 0 0.471292 1 1 1 1
  spline S77 degree 3 poles (-141.937, 27.9548) (-141.9087, 27.9475) (-141.8352, 27.9286) (-141.7591, 27.9291) (-141.7124, 27.9295) knots 0 0 0 0 0.385917 1 1 1 1
  line L280 (-141.7124, 27.9295) -> (-140.0874, 27.9295)
  spline S78 degree 3 poles (-140.0874, 27.9295) (-140.0059, 27.9288) (-139.8816, 27.9279) (-139.7579, 27.9392) (-139.7154, 27.9431) knots 0 0 0 0 0.656122 1 1 1 1
  spline S79 degree 3 poles (-139.7154, 27.9431) (-139.6951, 27.9474) (-139.6599, 27.9547) (-139.6323, 27.9774) (-139.6206, 27.9871) knots 0 0 0 0 0.576682 1 1 1 1
  spline S80 degree 3 poles (-139.6206, 27.9871) (-139.6132, 27.9982) (-139.5977, 28.0215) (-139.5961, 28.0495) (-139.5952, 28.0642) knots 0 0 0 0 0.476649 1 1 1 1
  spline S81 degree 3 poles (-139.5952, 28.0642) (-139.5971, 28.0836) (-139.6013, 28.128) (-139.6174, 28.1697) (-139.6265, 28.1931) knots 0 0 0 0 0.436566 1 1 1 1
  line L281 (-139.6265, 28.1931) -> (-139.5581, 28.2263)
  line L282 (-139.5581, 28.2263) -> (-139.3394, 27.6931)
  line L283 (-139.3394, 27.6931) -> (-139.3394, 27.6052)
  line L284 (-142.1167, 45.5291) -> (-142.1167, 46.2361)
  line L285 (-142.1167, 46.2361) -> (-140.8784, 47.1326)
  spline S82 degree 3 poles (-140.8784, 47.1326) (-140.8796, 47.1627) (-140.8816, 47.2167) (-140.8821, 47.2708) (-140.8823, 47.2947) knots 0 0 0 0 0.557334 1 1 1 1
  spline S83 degree 3 poles (-140.8823, 47.2947) (-140.8823, 47.3035) (-140.8822, 47.3217) (-140.8817, 47.3399) (-140.8814, 47.3494) knots 0 0 0 0 0.482063 1 1 1 1
  spline S84 degree 3 poles (-140.8814, 47.3494) (-140.881, 47.3593) (-140.8802, 47.3795) (-140.879, 47.3997) (-140.8784, 47.4099) knots 0 0 0 0 0.491762 1 1 1 1
  line L286 (-140.8784, 47.4099) -> (-141.648, 47.4099)
  spline S85 degree 3 poles (-141.648, 47.4099) (-141.7169, 47.4116) (-141.8249, 47.4142) (-141.923, 47.3709) (-141.9585, 47.3552) knots 0 0 0 0 0.637589 1 1 1 1
  spline S86 degree 3 poles (-141.9585, 47.3552) (-141.9835, 47.3257) (-142.0377, 47.2619) (-142.0421, 47.1778) (-142.0445, 47.1326) knots 0 0 0 0 0.461812 1 1 1 1
  line L287 (-142.0445, 47.1326) -> (-142.0445, 47.0291)
  line L288 (-142.0445, 47.0291) -> (-142.1167, 47.0291)
  line L289 (-142.1167, 47.0291) -> (-142.1167, 48.1638)
  line L290 (-142.1167, 48.1638) -> (-142.0445, 48.1638)
  line L291 (-142.0445, 48.1638) -> (-142.0445, 48.0642)
  spline S87 degree 3 poles (-142.0445, 48.0642) (-142.0414, 48.0133) (-142.0357, 47.9185) (-141.9669, 47.8539) (-141.9351, 47.824) knots 0 0 0 0 0.536984 1 1 1 1
  spline S88 degree 3 poles (-141.9351, 47.824) (-141.9013, 47.8122) (-141.8089, 47.78) (-141.7105, 47.7818) (-141.648, 47.783) knots 0 0 0 0 0.36511 1 1 1 1
  line L292 (-141.648, 47.783) -> (-139.937, 47.783)
  spline S89 degree 3 poles (-139.937, 47.783) (-139.8681, 47.7813) (-139.7601, 47.7787) (-139.662, 47.822) (-139.6265, 47.8377) knots 0 0 0 0 0.637589 1 1 1 1
  spline S90 degree 3 poles (-139.6265, 47.8377) (-139.6015, 47.8678) (-139.5473, 47.9331) (-139.5429, 48.0184) (-139.5405, 48.0642) knots 0 0 0 0 0.461715 1 1 1 1
  line L293 (-139.5405, 48.0642) -> (-139.5405, 48.1638)
  line L294 (-139.5405, 48.1638) -> (-139.4683, 48.1638)
  line L295 (-139.4683, 48.1638) -> (-139.4683, 47.199)
  spline S91 degree 3 poles (-139.4683, 47.199) (-139.4686, 47.0763) (-139.469, 46.8667) (-139.512, 46.6618) (-139.5298, 46.5769) knots 0 0 0 0 0.585417 1 1 1 1
  spline S92 degree 3 poles (-139.5298, 46.5769) (-139.5549, 46.5125) (-139.6054, 46.3826) (-139.7058, 46.2859) (-139.7564, 46.2371) knots 0 0 0 0 0.49578 1 1 1 1
  spline S93 degree 3 poles (-139.7564, 46.2371) (-139.8146, 46.1963) (-139.9328, 46.1136) (-140.0768, 46.1029) (-140.1499, 46.0974) knots 0 0 0 0 0.492399 1 1 1 1
  spline S94 degree 3 poles (-140.1499, 46.0974) (-140.2285, 46.1039) (-140.3849, 46.1169) (-140.511, 46.2102) (-140.5738, 46.2566) knots 0 0 0 0 0.50233 1 1 1 1